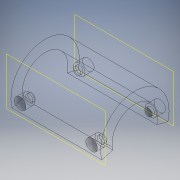
# Autodesk Inventor part: Slider Mount
Saved by Autodesk Inventor 2018 (Build 220112000, 112)
## iProperties
Created: 2018-01-05
Part Number: Slider Mount
Material: Generic
Document SubType Name: Modeling
Designer: njcfu
Density: 1 g/cm^3
Appearance: Default
Author: njcfu
Autodesk Inventor part; units mm, degrees
ref_plane "YZ Plane" through (0, 0, 0) normal (1, 0, 0) x (0, 1, 0)
ref_plane "XZ Plane" through (0, 0, 0) normal (0, 1, 0) x (-1, 0, 0)
sketch "Sketch1" plane through (0, 0, 0) normal (1, 0, 0) x (0, 1, 0)
  arc A0 (-4.9305, -18.4009) -> (-4.9305, 18.4009) centre (0, 0) ccw
  arc A1 (-3.287, -12.2673) -> (-3.287, 12.2673) centre (0, 0) ccw
  line L0 (-4.9305, 18.4009) -> (-3.287, 12.2673)
  line L1 (-3.287, -12.2673) -> (-4.9305, -18.4009)
  line L2 (0, 26.67) -> (0, -26.67) projected
  dimension "d0" = 19.05
  dimension "d1" = 12.7
  dimension "d5" = 6.35
  dimension "d6" = 6.35
  dimension "d7" = 15
  dimension "d8" = 15
  constraints: 5 point on circle, 4 end point, 2 centre point, 2 coincident
  measures "d0" radius of A0
  measures "d1" radius of A1
  measures "d5" distance of L1.start L1.end
  measures "d6" distance of L0.start L0.end
  measures "d7" angle of L2 L0
  measures "d8" angle of L2 L1
extrude "Extrusion1" add sketch "Sketch1" along normal mid plane 49.9999 contours L1 A1 L2 A0 | L2 A1 A0 | L2 A1 L0 A0
ref_plane "Work Plane2" through (0, 0, -19.05) normal (0, 0, 1) x (1, 0, 0)
sketch "Sketch10" plane through (0, 0, -19.05) normal (0, 0, 1) x (1, 0, 0)
  circle A0 centre (19.92, 0) radius 3.175
  circle A1 centre (-19.92, 0) radius 3.175
  line L0 (25, -4.9305) -> (25, 19.05) projected
  line L1 (-25, 19.05) -> (-25, -4.9305) projected
  line L2 (25, -4.9305) -> (-25, -4.9305) projected
  point P0 (0, 0)
  dimension "d62" = 5.08
  dimension "d63" = 5.08
  dimension "d64" = 4.9305
  dimension "d65" = 4.9305
  dimension "d66" = 6.35
  dimension "d67" = 6.35
  constraints: 2 centre point
  measures "d62" distance from line of L0 A0.centre
  measures "d63" distance from line of L1 A1.centre
  measures "d64" distance from line of L2 A1.centre
  measures "d65" distance from line of L2 A0.centre
  measures "d66" diameter of A0
  measures "d67" diameter of A1
extrude "Extrusion7" cut sketch "Sketch10" along normal blind 5.08
ref_plane "Work Plane3" through (0, 0, 19.05) normal (0, 0, 1) x (1, 0, 0)
sketch "Sketch11" plane through (0, 0, 19.05) normal (0, 0, 1) x (1, 0, 0)
  circle A0 centre (-19.92, 0) radius 3.175
  circle A1 centre (19.92, 0) radius 3.175
  line L0 (-25, 19.05) -> (-25, -4.9305) projected
  line L1 (25, -4.9305) -> (25, 19.05) projected
  line L2 (-25, -4.9305) -> (25, -4.9305) projected
  point P0 (0, 0)
  dimension "d70" = 5.08
  dimension "d71" = 5.08
  dimension "d72" = 6.35
  dimension "d73" = 6.35
  dimension "d74" = 4.9305
  dimension "d75" = 4.9305
  constraints: 2 centre point
  measures "d70" distance from line of L0 A0.centre
  measures "d71" distance from line of L1 A1.centre
  measures "d72" diameter of A0
  measures "d73" diameter of A1
  measures "d74" distance from line of L2 A1.centre
  measures "d75" distance from line of L2 A0.centre
extrude "Extrusion8" cut sketch "Sketch11" against normal blind 5.08
sketch "Sketch12" plane through (0, 0, 0) normal (0, 0, 1) x (1, 0, 0)
  circle A0 centre (-19.92, 0) radius 2.032
  circle A1 centre (19.92, 0) radius 2.032
  line L0 (-25, -4.9305) -> (25, -4.9305) projected
  line L1 (-25, 19.05) -> (-25, -4.9305) projected
  line L2 (25, -4.9305) -> (25, 19.05) projected
  point P0 (0, 0)
  dimension "d78" = 4.064
  dimension "d79" = 4.064
  dimension "d80" = 4.9305
  dimension "d81" = 4.9305
  dimension "d82" = 5.08
  dimension "d83" = 5.08
  constraints: 2 centre point
  measures "d78" diameter of A0
  measures "d79" diameter of A1
  measures "d80" distance from line of L0 A1.centre
  measures "d81" distance from line of L0 A0.centre
  measures "d82" distance from line of L1 A0.centre
  measures "d83" distance from line of L2 A1.centre
extrude "Extrusion9" cut sketch "Sketch12" along normal mid plane 50.8
body "Solid1"
